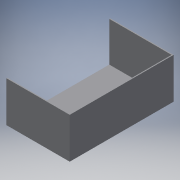
# Autodesk Inventor part: Part5
Saved by Autodesk Inventor 2016 (Build 200138000, 138)
## iProperties
Created: 2016-09-10
Part Number: Part5
Material: Generic
Document SubType Name: Modeling
Designer: gus
Density: 1 g/cm^3
Appearance: Default
Author: gus
Autodesk Inventor part; units mm, degrees
ref_plane "YZ Plane" through (0, 0, 0) normal (1, 0, 0) x (0, 1, 0)
ref_plane "XZ Plane" through (0, 0, 0) normal (0, 1, 0) x (-1, 0, 0)
ref_plane "XY Plane" through (0, 0, 0) normal (0, 0, 1) x (1, 0, 0)
sketch "Sketch1" plane through (0, 0, 0) normal (0, 1, 0) x (-1, 0, 0)
  line L0 (0, 0) -> (-177.8, 0)
  line L1 (-177.8, 0) -> (-177.8, -333.375)
  line L2 (-177.8, -333.375) -> (0, -333.375)
  line L3 (0, -333.375) -> (0, 0)
  dimension "d0" = 177.8
  dimension "d1" = 333.375
  constraints: 8 end point, 2 parallel, 1 horizontal, 1 perpendicular
  measures "d0" distance of L1.end L2.end
  measures "d1" distance of L0.end L1.end
extrude "Extrusion1" add sketch "Sketch1" along normal blind 3.175
sketch "Sketch2" plane through (0, 3.175, 0) normal (0, 1, 0) x (1, 0, 0)
  line L0 (0, 333.375) -> (0, 0) construction
  line L1 (0, 3.175) -> (174.625, 3.175)
  line L2 (174.625, 3.175) -> (174.625, 330.2)
  line L3 (174.625, 330.2) -> (0, 330.2)
  line L4 (177.8, 333.375) -> (0, 333.375) projected
  line L5 (177.8, 0) -> (177.8, 333.375) projected
  line L6 (0, 0) -> (177.8, 0) projected
  line L7 (0, 0) -> (0, 3.175)
  line L8 (0, 330.2) -> (0, 333.375)
  dimension "d4" = 3.175
  dimension "d5" = 3.175
  dimension "d6" = 3.175
  constraints: 10 end point, 3 perpendicular, 2 point on line, 1 collinear, 1 horizontal
  measures "d4" distance between parallel lines of L4 L3
  measures "d5" distance between parallel lines of L5 L2
  measures "d6" distance between parallel lines of L6 L1
extrude "Extrusion2" add sketch "Sketch2" along normal blind 127
body "Solid1"
